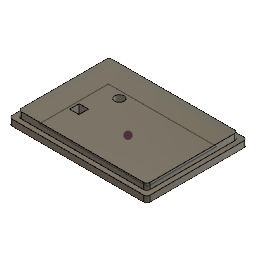
Light project lid v3 (Autodesk Fusion 360 design; units mm, degrees)
Autodesk Fusion 360 part; units mm, degrees
sketch "Sketch1" plane through (0, 0, 0) normal (0, 1, 0) x (1, 0, 0) in component "Lid"
sketch "Sketch2" plane through (0, 0, 0) normal (0, 1, 0) x (1, 0, 0) in component "Lid"
sketch "Sketch3" plane through (0, 0, 0) normal (0, 1, 0) x (1, 0, 0) in component "Lid"
  line L0 (55.88, 40.64) -> (-55.88, 40.64)
  line L1 (-55.88, 40.64) -> (-55.88, -40.64)
  line L2 (-55.88, -40.64) -> (55.88, -40.64)
  line L3 (55.88, -40.64) -> (55.88, 40.64)
  line L4 (55.88, 40.64) -> (-55.88, -40.64) construction
  line L5 (-55.88, 40.64) -> (55.88, -40.64) construction
  dimension "d1" = 111.76
  dimension "d2" = 81.28
extrude "Extrude1" add sketch "Sketch3" along normal blind 5.08 in component "Lid"
sketch "Sketch4" plane through (0, 5.08, 0) normal (0, 1, 0) x (-1, 0, 0) in component "Lid"
  line L0 (-55.88, 40.64) -> (-55.88, -40.64)
  line L1 (-55.88, -40.64) -> (55.88, -40.64)
  line L2 (55.88, -40.64) -> (55.88, 40.64)
  line L3 (55.88, 40.64) -> (-55.88, 40.64)
  line L4 (-52.07, -36.83) -> (52.07, -36.83)
  line L5 (52.07, -36.83) -> (52.07, 36.83)
  line L6 (52.07, 36.83) -> (-52.07, 36.83)
  line L7 (-52.07, 36.83) -> (-52.07, -36.83)
  line L8 (-52.07, -36.83) -> (52.07, 36.83) construction
  line L9 (52.07, -36.83) -> (-52.07, 36.83) construction
  dimension "d5" = 104.14
  dimension "d6" = 73.66
extrude "Extrude2" add sketch "Sketch4" along normal blind 5.08 contours L4 L5 L6 L7 in component "Lid"
fillet "Fillet1" radius 2.54 8 edges at (52.07, 7.62, 36.83) (-52.07, 7.62, 36.83) (52.07, 7.62, -36.83) (-52.07, 7.62, -36.83) (-55.88, 2.54, -40.64) (55.88, 2.54, -40.64) (55.88, 2.54, 40.64) (-55.88, 2.54, 40.64) in component "Lid"
sketch "Sketch1 (2)" plane through (0, 0, 0) normal (0, -1, 0) x (1, 0, 0)
  arc A0 (-53.34, 40.64) -> (-55.88, 38.1) centre (-53.34, 38.1) ccw
  line L0 (-55.88, 38.1) -> (-55.88, -38.1)
  arc A1 (-55.88, -38.1) -> (-53.34, -40.64) centre (-53.34, -38.1) ccw
  line L1 (-53.34, -40.64) -> (53.34, -40.64)
  arc A2 (53.34, -40.64) -> (55.88, -38.1) centre (53.34, -38.1) ccw
  line L2 (55.88, -38.1) -> (55.88, 38.1)
  arc A3 (55.88, 38.1) -> (53.34, 40.64) centre (53.34, 38.1) ccw
  line L3 (53.34, 40.64) -> (-53.34, 40.64)
  line L4 (43.815, 27.94) -> (-43.815, 27.94)
  line L5 (-43.815, 27.94) -> (-43.815, -27.94)
  line L6 (-43.815, -27.94) -> (43.815, -27.94)
  line L7 (43.815, -27.94) -> (43.815, 27.94)
  line L8 (43.815, 27.94) -> (-43.815, -27.94) construction
  line L9 (-43.815, 27.94) -> (43.815, -27.94) construction
  dimension "d10" = 87.63
  dimension "d11" = 55.88
sketch "Sketch2 (2)" plane through (0, 0, 0) normal (0, -1, 0) x (1, 0, 0)
  circle A0 centre (-19.05, -12.065) radius 3.81
  dimension "d12" = 7.62
  dimension "d13" = 24.765
  dimension "d14" = 15.875
  measures "d12" diameter of A0
  measures "d13" distance of origin
  measures "d14" distance of origin
extrude "Extrude3" cut sketch "Sketch2 (2)" against normal blind 10.16 in component "Lid"
sketch "Sketch3 (2)" plane through (0, 0, 0) normal (0, 1, 0) x (1, 0, 0)
  line L0 (-24.13, -15.494) -> (-31.75, -15.494)
  line L1 (-31.75, -15.494) -> (-31.75, -7.874)
  line L2 (-31.75, -7.874) -> (-24.13, -7.874)
  line L3 (-24.13, -7.874) -> (-24.13, -15.494)
  line L4 (-24.13, -15.494) -> (-31.75, -7.874) construction
  line L5 (-31.75, -15.494) -> (-24.13, -7.874) construction
  dimension "d17" = 7.62
  dimension "d18" = 7.62
  dimension "d19" = 39.624
  dimension "d20" = 15.875
  measures "d19" distance of origin
  measures "d20" distance of origin
extrude "Extrude4" cut sketch "Sketch3 (2)" along normal blind 10.16 in component "Lid"
component "Lid" placed x (1, 0, 0) y (0, 1, 0) z (0, 0, 1) at (0, 0, 0)
